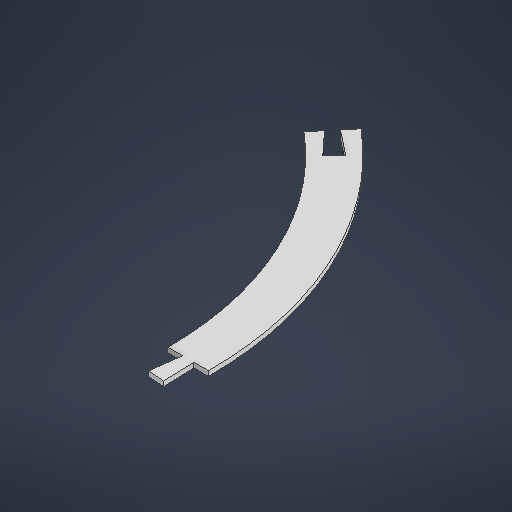
# Autodesk Inventor part: base
Saved by Autodesk Inventor 2026.2 (Build 302298000, 298)
## iProperties
Created: 2026-02-13
Part Number: base
Material: Genérico
Document SubType Name: Chapa de metal
Designer: Ian
Density: 1 g/cm^3
Appearance: Padrão
Sheet Metal Rule: Padrão
Author: Ian
Autodesk Inventor part; units mm, degrees
ref_plane "YZ Plane" through (0, 0, 0) normal (1, 0, 0) x (0, 1, 0)
ref_plane "XZ Plane" through (0, 0, 0) normal (0, 1, 0) x (-1, 0, 0)
ref_plane "XY Plane" through (0, 0, 0) normal (0, 0, 1) x (1, 0, 0)
sketch "Esboço1" plane through (0, 0, 0) normal (0, 1, 0) x (-1, 0, 0)
  arc A0 (-410, 0) -> (-289.9138, -289.9138) centre (0, 0) ccw
  arc A1 (-460, 0) -> (-325.2691, -325.2691) centre (0, 0) ccw
  circle A2 centre (0, 0) radius 460
  circle A3 centre (0, 0) radius 410
  line L0 (0, 0) -> (-407.9373, -407.9373)
  line L1 (0, 0) -> (-1224.3013, 0) construction
  line L2 (-410, 0) -> (-460, 0)
  point P0 (-460, 0)
  point P1 (-325.2691, -325.2691)
  point P2 (-289.9138, -289.9138)
  dimension "d27" = 820
  dimension "d28" = 920
  dimension "d87" = 45
  constraints: 6 end point, 6 point on circle, 4 coincident, 3 centre point, 1 horizontal, 1 horizontal alignment, 3 other
  measures "d27" diameter of A0
  measures "d28" diameter of A1
  measures "d87" angle of L1 L0
extrude "Extrusão1" add sketch "Esboço1" along normal blind 6 contours A0 L0 A1 L2
sketch "Esboço6" plane through (0, 6, 0) normal (0, 1, 0) x (1, 0, 0)
  arc A0 (460, 0) -> (325.2691, 325.2691) centre (0, 0) ccw projected
  circle A1 centre (0, 0) radius 460
  arc A2 (410, 0) -> (289.9138, 289.9138) centre (0, 0) ccw projected
  circle A3 centre (0, 0) radius 410
  line L0 (0, 0) -> (743.005, -65.0045)
  line L1 (410, 0) -> (460, 0) projected
  line L2 (410, 0) -> (428, 0)
  line L3 (428, 0) -> (442, 0)
  line L4 (408.4398, -35.7339) -> (423.3827, -37.0412)
  line L5 (423.3827, -37.0412) -> (443.3066, -38.7843)
  line L6 (428, 0) -> (423.3827, -37.0412)
  line L7 (442, 0) -> (443.3066, -38.7843)
  dimension "d110" = 5
  dimension "d111" = 18
  dimension "d112" = 14
  dimension "d113" = 15
  dimension "d114" = 20
  constraints: 14 end point, 5 point on line, 2 point on circle, 1 centre point, 1 coincident, 1 horizontal alignment, 2 other
  measures "d110" angle of L1 L0
  measures "d111" distance of L1.start L2.end
  measures "d112" distance of L2.end L3.end
  measures "d113" distance of L4.start L4.end
  measures "d114" distance of L4.end L5.end
extrude "Extrusão6" add sketch "Esboço6" against normal up to surface (6 mm away) contours L7 L0 L6 L1
sketch "Esboço8" plane through (0, 6, 0) normal (0, 1, 0) x (1, 0, 0)
  arc A0 (325.2691, 325.2691) -> (295.6823, 352.3804) centre (0, 0) ccw
  arc A1 (289.9138, 289.9138) -> (263.5429, 314.0782) centre (0, 0) ccw
  line L0 (0, 0) -> (410.9037, 489.696)
  line L1 (325.2691, 325.2691) -> (289.9138, 289.9138) projected
  line L2 (325.2691, 325.2691) -> (314.6625, 314.6625)
  line L3 (314.6625, 314.6625) -> (300.5204, 300.5204)
  line L4 (295.6823, 352.3804) -> (284.1121, 338.5916)
  line L5 (284.1121, 338.5916) -> (275.1131, 327.867)
  line L6 (275.1131, 327.867) -> (300.5204, 300.5204)
  line L7 (284.1121, 338.5916) -> (314.6625, 314.6625)
  dimension "d130" = 5
  dimension "d131" = 15
  dimension "d132" = 20
  dimension "d133" = 18
  dimension "d134" = 14
  constraints: 15 end point, 6 point on line, 4 point on circle, 2 centre point, 2 coincident
  measures "d130" angle of L1 L0
  measures "d131" distance of L1.start L2.end
  measures "d132" distance of L2.end L3.end
  measures "d133" distance of L4.start L4.end
  measures "d134" distance of L4.end L5.end
extrude "Extrusão7" add sketch "Esboço8" against normal blind 10 contours L1 L7 L0 A0 | L1 A1 L0 L6
equation "\"Raio_vergadura\" = Espessura"
equation "\"Largura_alívio_de_vergadura\" = Espessura"
equation "\"Profundidade_alívio_de_vergadura\" = 0.5 * Espessura"
equation "\"Tamanho_alívio_de_dobra\" = 4 * Espessura"
equation "\"Remanescente_mínimo\" = 2 * Espessura"
equation "\"Raiodetransição\" = Raio_vergadura"
equation "\"Tamanho_de_raio_de_Jacobi\" = Raio_vergadura"
equation "\"TamanhoFolga\" = Espessura"
equation "\"Espessura\" = 3.048"
